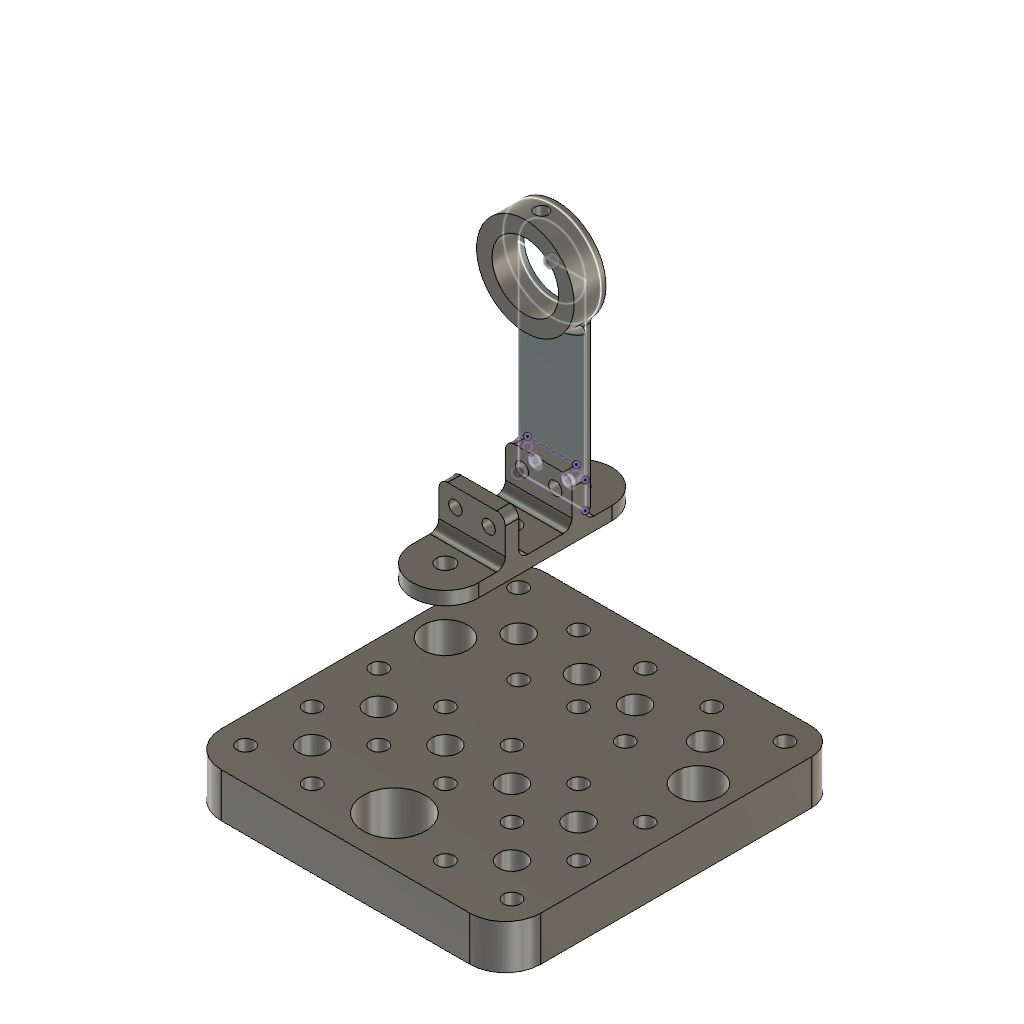
kobra2-neo-pen-holder (Autodesk Fusion 360 design; units mm, degrees)
Autodesk Fusion 360 part; units mm, degrees
note: some values were not read from the file. Chosen so that the rebuilt part matches the saved one: that a step has no effect; which face or edge a step refers to. Set by a fixed rule: which sketch regions a step uses.
sketch "Plate_Base_Profile" plane through (0, 0, 0) normal (0, 0, 1) x (1, 0, 0)
  line L0 (0, 0) -> (30, 0) construction
  circle A0 centre (30, 0) radius 1.9
  line L1 (0, 150) -> (0, -150) construction
  line L2 (0, 0) -> (0, -18) construction
  line L3 (0, -18) -> (12, -18) construction
  circle A1 centre (12, -18) radius 1.9
  line L4 (0, 0) -> (28.5, 0) construction
  line L5 (28.5, 0) -> (28.5, -18) construction
  circle A2 centre (28.5, -18) radius 5
  line L6 (0, 0) -> (0, -58) construction
  circle A3 centre (0, -58) radius 7
  circle A4 centre (0, -58) radius 11 construction
  circle A5 centre (30, 0) radius 6
  line L7 (30, 0) -> (30, 6) construction
  line L8 (30, 0) -> (36, 0) construction
  line L9 (30, 6) -> (0, 6)
  line L10 (0, -69) -> (28, -69)
  line L11 (36, 0) -> (36, -61)
  circle A6 centre (0, -58) radius 7
  line L12 (-30, 0) -> (-30, 6) construction
  circle A7 centre (-12, -18) radius 1.9
  circle A8 centre (-30, 0) radius 6
  line L13 (-30, 6) -> (0, 6)
  line L14 (0, 0) -> (-30, 0) construction
  circle A9 centre (0, -58) radius 11 construction
  line L15 (0, -69) -> (-28, -69)
  circle A10 centre (-30, 0) radius 1.9
  line L16 (0, 0) -> (-28.5, 0) construction
  line L17 (-28.5, 0) -> (-28.5, -18) construction
  circle A11 centre (-28.5, -18) radius 5
  line L18 (0, 0) -> (0, -18) construction
  line L19 (-36, 0) -> (-36, -61)
  line L20 (0, 0) -> (0, -58) construction
  line L21 (0, -18) -> (-12, -18) construction
  line L22 (-30, 0) -> (-36, 0) construction
  arc A12 (-36, -61) -> (-28, -69) centre (-28, -61) ccw
  arc A13 (28, -69) -> (36, -61) centre (28, -61) ccw
  dimension "d1" = 30
  dimension "d2" = 3.8
  dimension "d3" = 300
  dimension "d4" = 18
  dimension "d5" = 12
  dimension "d6" = 3.8
  dimension "d7" = 28.5
  dimension "d8" = 18
  dimension "d9" = 10
  dimension "d10" = 58
  dimension "d11" = 14
  dimension "d12" = 22
  dimension "d13" = 12
  dimension "d14" = 8
  constraint coincident L0.start L2.start
  constraint horizontal L0
  constraint coincident L0.end A0.centre
  constraint vertical L1
  constraint perpendicular L0 L2
  constraint perpendicular L2 L3
  constraint coincident L3.end A1.centre
  constraint perpendicular L1 L4
  constraint perpendicular L0 L5
  constraint coincident L5.end A2.centre
  constraint perpendicular L4 L6
  constraint coincident L6.end A3.centre
  constraint concentric A3 A4
  constraint concentric A0 A5
  constraint coincident A5 L7.end
  constraint perpendicular L0 L7
  constraint coincident A5 L8.end
  constraint perpendicular L7 L8
  constraint coincident L1 L9.end
  constraint tangent A5 L9
  constraint coincident A4 L10.start
  constraint coincident L1 L10.start
  constraint tangent A4 L10
  constraint perpendicular L1 L10
  constraint tangent A5 L11
  constraint symmetric L0.start L1 L2.start
  constraint symmetric L0.end L1 L12.start
  constraint symmetric A0 L1 A10
  constraint symmetric L1 L2.end L3.start
  constraint symmetric L1 L3.end A7.centre
  constraint symmetric L1 A1 A7
  constraint symmetric L1 L4.end L16.end
  constraint symmetric L1 L5.end L17.end
  constraint symmetric L1 A2 A11
  constraint symmetric L1 L6.end A3.centre
  constraint symmetric L1 A3 A6
  constraint symmetric L1 A4 A9
  constraint symmetric L1 A5 A8
  constraint symmetric L1 L7.end L12.end
  constraint symmetric L1 L8.end L19.start
  constraint symmetric L1 L9.end L13.end
  constraint symmetric L1 L10.start L15.start
  constraint tangent L19 A12
  constraint tangent L15 A12
  constraint tangent L10 A13
  constraint tangent L11 A13
  constraint equal A12 A13
  constraint tangent A4 L15
  constraint tangent A8 L19
  constraint midpoint L0.start L1
  measures "d1" distance of L0.start L0.end
  measures "d2" diameter of A0
  measures "d3" distance of L1.start L1.end
  measures "d4" distance of L0.start L2.end
  measures "d5" distance of L2.end L3.end
  measures "d6" diameter of A1
  measures "d7" distance of L0.start L4.end
  measures "d8" distance of L4.end L5.end
  measures "d9" diameter of A2
  measures "d10" distance of L0.start L6.end
  measures "d11" diameter of A3
  measures "d12" diameter of A4
  measures "d13" diameter of A5
  measures "d14" radius of A12
extrude "Plate_Base" add sketch "Plate_Base_Profile" along normal blind 10 makes body 1
sketch "Grid_Hole_Seed" plane through (0, 0, 10) normal (0, 0, 1) x (-1, 0, 0)
  circle A0 centre (28.5, 18) radius 5
  circle A1 centre (-30, 0) radius 1.9
  circle A2 centre (30, 0) radius 1.9
  circle A3 centre (12, 18) radius 1.9
  circle A4 centre (0, 58) radius 7
  circle A5 centre (-28.5, 18) radius 5
  circle A6 centre (-12, 18) radius 1.9
  line L0 (28, 69) -> (-28, 69)
  arc A7 (-28, 69) -> (-36, 61) centre (-28, 61) ccw
  line L1 (-36, 61) -> (-36, 0)
  arc A8 (-36, 0) -> (-30, -6) centre (-30, 0) ccw
  line L2 (-30, -6) -> (30, -6)
  arc A9 (30, -6) -> (36, 0) centre (30, 0) ccw
  line L3 (36, 0) -> (36, 61)
  arc A10 (36, 61) -> (28, 69) centre (28, 61) ccw
  line L4 (0, -6) -> (0, 69) construction
  circle A11 centre (0, 31.5) radius 1.9
  dimension "d19" = 3.8
  constraint midpoint L2 L4.start
  constraint coincident L0 L4.end
  constraint perpendicular L0 L4
  constraint midpoint L4 A11.centre
  measures "d19" diameter of A11
extrude "Grid_Hole_Cut" cut sketch "Grid_Hole_Seed" against normal through all contours A11 bodies 1
pattern_linear "Grid_Hole_Pattern" [no effect]
sketch "Mounting_Holes" plane through (0, 0, 10) normal (0, 0, 1) x (-1, 0, 0)
  circle A0 centre (0, 31.5) radius 1.9
  circle A1 centre (28.5, 18) radius 5
  circle A2 centre (-30, 0) radius 1.9
  circle A3 centre (30, 0) radius 1.9
  circle A4 centre (12, 18) radius 1.9
  circle A5 centre (0, 58) radius 7
  circle A6 centre (-28.5, 18) radius 5
  circle A7 centre (-12, 18) radius 1.9
  line L0 (28, 69) -> (-28, 69)
  arc A8 (-28, 69) -> (-36, 61) centre (-28, 61) ccw
  line L1 (-36, 61) -> (-36, 0)
  arc A9 (-36, 0) -> (-30, -6) centre (-30, 0) ccw
  line L2 (-30, -6) -> (30, -6)
  arc A10 (30, -6) -> (36, 0) centre (30, 0) ccw
  line L3 (36, 0) -> (36, 61)
  arc A11 (36, 61) -> (28, 69) centre (28, 61) ccw
  circle A12 centre (-30, 61.5) radius 1.9
  circle A13 centre (-30, 46.5) radius 1.9
  circle A14 centre (-30, 31.5) radius 1.9
  circle A15 centre (-15, 61.5) radius 1.9
  circle A16 centre (-15, 46.5) radius 1.9
  circle A17 centre (-15, 31.5) radius 1.9
  circle A18 centre (-15, 1.5) radius 1.9
  circle A19 centre (0, 46.5) radius 1.9
  circle A20 centre (0, 16.5) radius 1.9
  circle A21 centre (0, 1.5) radius 1.9
  circle A22 centre (15, 61.5) radius 1.9
  circle A23 centre (15, 46.5) radius 1.9
  circle A24 centre (15, 31.5) radius 1.9
  circle A25 centre (15, 1.5) radius 1.9
  circle A26 centre (30, 61.5) radius 1.9
  circle A27 centre (30, 46.5) radius 1.9
  circle A28 centre (30, 31.5) radius 1.9
  line L4 (15, 31.5) -> (30, 46.5) construction
  line L5 (30, 46.5) -> (30, 31.5) construction
  line L6 (30, 31.5) -> (15, 46.5) construction
  line L7 (15, 46.5) -> (0, 31.5) construction
  line L8 (0, 31.5) -> (-15, 46.5) construction
  line L9 (-15, 46.5) -> (-29.5655, 31.9345) construction
  line L10 (-29.5655, 31.9345) -> (-30, 46.5) construction
  line L11 (-30, 46.5) -> (-15, 31.5) construction
  line L12 (-15, 31.5) -> (0, 46.5) construction
  line L13 (0, 46.5) -> (15, 31.5) construction
  line L14 (0, 1.5) -> (12, 18) construction
  line L15 (0, 1.5) -> (-12, 18) construction
  line L16 (-12, 18) -> (-30, 0) construction
  line L17 (12, 18) -> (30, 0) construction
  line L18 (30, 46.5) -> (30, 61.5) construction
  line L19 (30, 61.5) -> (15, 46.5) construction
  line L20 (30, 46.5) -> (15, 61.5) construction
  line L21 (-15, 61.5) -> (-30, 46.5) construction
  line L22 (-30, 61.5) -> (-15, 46.5) construction
  circle A29 centre (22.5, 39) radius 3
  circle A30 centre (7.5, 39) radius 3
  circle A31 centre (-7.5, 39) radius 3
  circle A32 centre (-22.5, 39) radius 3
  circle A33 centre (22.5, 54) radius 3
  circle A34 centre (-22.5, 54) radius 3
  circle A35 centre (21, 9) radius 3
  circle A36 centre (6, 9.75) radius 3
  circle A37 centre (-6, 9.75) radius 3
  circle A38 centre (-21, 9) radius 3
  dimension "d26" = 6
  dimension "d27" = 6
  dimension "d28" = 6
  dimension "d29" = 6
  dimension "d30" = 6
  dimension "d31" = 6
  dimension "d32" = 6
  dimension "d33" = 6
  dimension "d34" = 6
  dimension "d35" = 6
  constraint coincident A24.centre L4.start
  constraint coincident A27.centre L4.end
  constraint coincident A28.centre L5.end
  constraint coincident A23.centre L6.end
  constraint coincident A0.centre L7.end
  constraint coincident A16.centre L8.end
  constraint perpendicular L8 L9
  constraint coincident A13.centre L10.end
  constraint coincident A17.centre L11.end
  constraint coincident A19.centre L12.end
  constraint coincident A21.centre L14.start
  constraint coincident A4.centre L14.end
  constraint coincident A7.centre L15.end
  constraint coincident A2.centre A9.centre
  constraint coincident A3.centre A10.centre
  constraint coincident A26.centre L18.end
  constraint coincident A22.centre L20.end
  constraint coincident A15.centre L21.start
  constraint coincident A12.centre L22.start
  constraint midpoint L4 A29.centre
  constraint midpoint L13 A30.centre
  constraint midpoint L12 A31.centre
  constraint midpoint L11 A32.centre
  constraint midpoint L19 A33.centre
  constraint midpoint L21 A34.centre
  constraint midpoint L17 A35.centre
  constraint midpoint L14 A36.centre
  constraint midpoint L15 A37.centre
  constraint midpoint L16 A38.centre
  measures "d26" diameter of A29
  measures "d27" diameter of A30
  measures "d28" diameter of A31
  measures "d30" diameter of A33
  measures "d32" diameter of A35
  measures "d33" diameter of A36
  measures "d34" diameter of A37
  measures "d35" diameter of A38
extrude "Mounting_Holes_Cut" cut sketch "Mounting_Holes" against normal through all contours A12 | A13 | A14 | A15 | A16 | A17 | A18 | A19 | A20 | A21 | A22 | A23 | A24 | A25 | A26 | A27 | A28 | A29 | A30 | A31 | A32 | A33 | A34 | A35 | A36 | A37 | A38 bodies 1
ref_plane "WorkPlane1" through (0, -31.5, 50) normal (0, 0, 1) x (1, 0, 0)
sketch "Pen_Base_Profile" plane through (0, 0, 50) normal (0, 0, 1) x (1, 0, 0)
  circle A0 centre (-30, -31.5) radius 1.9
  circle A1 centre (-30, -46.5) radius 1.9
  circle A2 centre (-30, -61.5) radius 1.9
  circle A3 centre (-15, -1.5) radius 1.9
  circle A4 centre (-15, -31.5) radius 1.9
  circle A5 centre (-15, -46.5) radius 1.9
  circle A6 centre (-15, -61.5) radius 1.9
  circle A7 centre (0, -1.5) radius 1.9
  circle A8 centre (0, -16.5) radius 1.9
  circle A9 centre (0, -46.5) radius 1.9
  circle A10 centre (15, -1.5) radius 1.9
  circle A11 centre (15, -31.5) radius 1.9
  circle A12 centre (15, -46.5) radius 1.9
  circle A13 centre (15, -61.5) radius 1.9
  circle A14 centre (30, -31.5) radius 1.9
  circle A15 centre (30, -46.5) radius 1.9
  circle A16 centre (30, -61.5) radius 1.9
  arc A17 (36, 0) -> (30, 6) centre (30, 0) ccw
  line L0 (30, 6) -> (-30, 6)
  arc A18 (-30, 6) -> (-36, 0) centre (-30, 0) ccw
  line L1 (-36, 0) -> (-36, -61)
  arc A19 (-36, -61) -> (-28, -69) centre (-28, -61) ccw
  line L2 (-28, -69) -> (28, -69)
  arc A20 (28, -69) -> (36, -61) centre (28, -61) ccw
  line L3 (36, -61) -> (36, 0)
  circle A21 centre (30, 0) radius 1.9
  circle A22 centre (-12, -18) radius 1.9
  circle A23 centre (-28.5, -18) radius 5
  circle A24 centre (28.5, -18) radius 5
  circle A25 centre (0, -58) radius 7
  circle A26 centre (12, -18) radius 1.9
  circle A27 centre (-30, 0) radius 1.9
  circle A28 centre (0, -31.5) radius 1.9
  circle A29 centre (-22.5, -54) radius 3
  circle A30 centre (22.5, -54) radius 3
  circle A31 centre (-6, -9.75) radius 3
  circle A32 centre (6, -9.75) radius 3
  circle A33 centre (7.5, -39) radius 3
  circle A34 centre (-22.5, -39) radius 3
  circle A35 centre (22.5, -39) radius 3
  circle A36 centre (-21, -9) radius 3
  circle A37 centre (21, -9) radius 3
  circle A38 centre (-7.5, -39) radius 3
  circle A39 centre (0, -16.5) radius 7.5
  circle A40 centre (0, -46.5) radius 7.5
  line L4 (0, -46.5) -> (-7.5, -46.5) construction
  line L5 (-7.5, -16.5) -> (0, -16.5) construction
  line L6 (-7.5, -16.5) -> (-7.5, -46.5)
  line L7 (0, -16.5) -> (7.5, -16.5) construction
  line L8 (0, -46.5) -> (7.5, -46.5) construction
  line L9 (7.5, -16.5) -> (7.5, -46.5)
  circle A41 centre (0, -16.5) radius 2
  circle A42 centre (0, -46.5) radius 2
  dimension "d62" = 15
  dimension "d63" = 15
  dimension "d64" = 4
  dimension "d65" = 4
  constraint concentric A8 A39
  constraint concentric A9 A40
  constraint coincident A9.centre A40.centre
  constraint coincident A40 L4.end
  constraint horizontal L4
  constraint coincident A39 L5.start
  constraint coincident A8.centre A39.centre
  constraint tangent A40 L6
  constraint coincident A39 L7.end
  constraint parallel L5 L7
  constraint coincident A40 L8.end
  constraint parallel L4 L8
  constraint concentric A8 A41
  constraint concentric A40 A42
  measures "d62" diameter of A39
  measures "d63" diameter of A40
  measures "d64" diameter of A41
  measures "d65" diameter of A42
extrude "Pen_Base_Plate" add sketch "Pen_Base_Profile" along normal blind 3 separate body contours A25 A40 | A25 A40 | A33 A38 A39 A40 L6 L9 | A33 L9 | A38 L6 | A31 A32 A39 | A32 A39 | A31 A39 picked at (0, -52.9878) picked at (-3.6256, -49.8497) picked at (6.2303, -39.7331) picked at (-5.9134, -39.6549) picked at (4.6509, -11.2678) picked at (-4.6663, -11.2812) makes body 2
sketch "Pen_Base_Reinforcements" plane through (0, 0, 53) normal (0, 0, 1) x (-1, 0, 0)
  circle A0 centre (0, 46.5) radius 2
  circle A1 centre (0, 16.5) radius 2
  circle A2 centre (0, 31.5) radius 1.9
  line L0 (7.5, 16.5) -> (7.5, 46.5)
  arc A3 (7.5, 46.5) -> (-7.5, 46.5) centre (0, 46.5) ccw
  line L1 (-7.5, 46.5) -> (-7.5, 16.5)
  arc A4 (-7.5, 16.5) -> (7.5, 16.5) centre (0, 16.5) ccw
  line L2 (0, 16.5) -> (0, 31.5) construction
  line L3 (0, 31.5) -> (0, 46.5) construction
  line L4 (0, 39) -> (7.5, 39) construction
  line L5 (0, 24) -> (7.5, 24) construction
  line L6 (0, 24) -> (-7.5, 24) construction
  line L7 (0, 39) -> (-7.5, 39) construction
  line L8 (-7.5, 40.5) -> (7.5, 40.5)
  line L9 (7.5, 40.5) -> (7.5, 37.5)
  line L10 (7.5, 37.5) -> (-7.5, 37.5)
  line L11 (-7.5, 37.5) -> (-7.5, 40.5)
  line L12 (-7.5, 40.5) -> (7.5, 37.5) construction
  line L13 (7.5, 40.5) -> (-7.5, 37.5) construction
  line L14 (-7.5, 25.5) -> (7.5, 25.5)
  line L15 (7.5, 25.5) -> (7.5, 22.5)
  line L16 (7.5, 22.5) -> (-7.5, 22.5)
  line L17 (-7.5, 22.5) -> (-7.5, 25.5)
  line L18 (-7.5, 25.5) -> (7.5, 22.5) construction
  line L19 (7.5, 25.5) -> (-7.5, 22.5) construction
  point P0 (0, 39)
  point P1 (0, 24)
  dimension "d68" = 3
  dimension "d69" = 3
  dimension "d119" = 15
  constraint coincident A1.centre A4.centre
  constraint coincident A2.centre L2.end
  constraint coincident A0.centre A3.centre
  constraint midpoint L3 P0
  constraint coincident L0 L4.end
  constraint perpendicular L0 L4
  constraint midpoint L2 P1
  constraint coincident L0 L5.end
  constraint perpendicular L0 L5
  constraint coincident L1 L6.end
  constraint perpendicular L1 L6
  constraint coincident L1 L7.end
  constraint perpendicular L1 L7
  constraint horizontal L8
  constraint perpendicular L8 L9
  constraint parallel L8 L10
  constraint parallel L9 L11
  constraint coincident L12 P0
  constraint coincident L13 P0
  constraint coincident P0 L4.start
  constraint horizontal L14
  constraint perpendicular L14 L15
  constraint parallel L14 L16
  constraint parallel L15 L17
  constraint coincident L18 P1
  constraint coincident L19 P1
  constraint coincident P1 L5.start
  constraint equal L8 L14
  measures "d68" distance of L8.end L9.end
  measures "d69" distance of L14.end L15.end
  measures "d119" horizontal distance of L8.start L8.end
extrude "Pen_Base_Reinforcement" add sketch "Pen_Base_Reinforcements" along normal blind 10 contours L0 L1 L14 L15 L16 L17 | L0 L1 L8 L9 L10 L11 bodies 2
fillet "Pen_Base_Fillet_A" radius 2 4 edges at (0, -22.5, 53) (0, -37.5, 53) (0, -25.5, 53) (0, -40.5, 53) on bodies 2
fillet "Pen_Base_Fillet_B" radius 2 4 edges at (-7.5, -24, 63) (7.5, -24, 63) (-7.5, -39, 63) (7.5, -39, 63) on bodies 2
sketch "Insert_Pilot_Holes" plane through (0, -22.5, 0) normal (0, 1, 0) x (-1, 0, 0)
  arc A0 (-5.5, 63) -> (-7.5, 61) centre (-5.5, 61) ccw
  line L0 (-7.5, 61) -> (-7.5, 55)
  line L1 (-7.5, 55) -> (7.5, 55)
  line L2 (7.5, 55) -> (7.5, 61)
  arc A1 (7.5, 61) -> (5.5, 63) centre (5.5, 61) ccw
  line L3 (5.5, 63) -> (-5.5, 63)
  line L4 (7.5, 53) -> (7.5, 55)
  line L5 (7.5, 55) -> (-7.5, 55)
  line L6 (-7.5, 55) -> (-7.5, 53)
  line L7 (-7.5, 53) -> (7.5, 53)
  line L8 (0, 53) -> (0, 63) construction
  line L9 (0, 55) -> (0, 59) construction
  line L10 (0, 59) -> (3.75, 59) construction
  line L11 (0, 59) -> (-3.75, 59) construction
  circle A2 centre (3.75, 59) radius 1.5
  circle A3 centre (-3.75, 59) radius 1.5
  dimension "d76" = 4
  dimension "d77" = 3.75
  dimension "d78" = 3.75
  dimension "d79" = 3
  dimension "d80" = 3
  constraint midpoint L7 L8.start
  constraint midpoint L3 L8.end
  constraint midpoint L5 L9.start
  constraint perpendicular L3 L9
  constraint perpendicular L2 L10
  constraint perpendicular L8 L11
  constraint coincident L10.end A2.centre
  constraint coincident L11.end A3.centre
  measures "d76" distance of L9.start L9.end
  measures "d77" distance of L9.end L10.end
  measures "d78" distance of L9.end L11.end
  measures "d79" diameter of A2
  measures "d80" diameter of A3
extrude "Insert_Pilot_Holes_Cut" cut sketch "Insert_Pilot_Holes" against normal up to surface (18 mm away) contours A2 | A3 bodies 2
sketch "Flex_Link_And_Pen_Clamp_Profile" plane through (0, -22.5, 0) normal (0, 1, 0) x (-1, 0, 0)
  arc A0 (-5.5, 63) -> (-7.5, 61) centre (-5.5, 61) ccw
  line L0 (-7.5, 61) -> (-7.5, 55)
  line L1 (-7.5, 55) -> (7.5, 55)
  line L2 (7.5, 55) -> (7.5, 61)
  arc A1 (7.5, 61) -> (5.5, 63) centre (5.5, 61) ccw
  line L3 (5.5, 63) -> (-5.5, 63)
  line L4 (7.5, 55) -> (-7.5, 55)
  line L5 (-7.5, 55) -> (-7.5, 100)
  line L6 (-7.5, 100) -> (7.5, 100)
  line L7 (7.5, 100) -> (7.5, 55)
  circle A2 centre (-3.75, 59) radius 1.3
  circle A3 centre (3.75, 59) radius 1.3
  circle A4 centre (0, 100) radius 11
  circle A5 centre (0, 100) radius 7.5
  circle A6 centre (3.75, 59) radius 1.5
  circle A7 centre (-3.75, 59) radius 1.5
  dimension "d83" = 15
  dimension "d84" = 45
  dimension "d85" = 2.6
  dimension "d86" = 2.6
  dimension "d87" = 22
  dimension "d121" = 15
  constraint horizontal L4
  constraint vertical L5
  constraint horizontal L6
  constraint vertical L7
  constraint coincident L1.end L2.start
  constraint midpoint L6 A4.centre
  constraint concentric A4 A5
  constraint concentric A2 A7
  constraint concentric A3 A6
  measures "d83" distance of L1.end L0.end
  measures "d84" distance of L1.end L6.end
  measures "d85" diameter of A2
  measures "d86" diameter of A3
  measures "d87" diameter of A4
  measures "d121" diameter of A5
extrude "Flex_Link_Base" add sketch "Flex_Link_And_Pen_Clamp_Profile" along normal blind 1.2 separate body contours A0 L0 L1 L2 A1 L3 L4 L5 L7 | A0 A1 L3 L5 L7 A4 | L5 L7 A4 A5 | L5 L7 A4 A5 | A6 | A7 makes body 3
extrude "Pen_Clamp_Reinforcement" add sketch "Flex_Link_And_Pen_Clamp_Profile" against normal blind 6 contours L5 L7 A4 A5 | L5 L7 A4 A5 bodies 3
fillet "Pen_Clamp_Fillet" radius 2 3 edges at (-7.5, -21.9, 91.9533) (0, -22.5, 89) (7.5, -21.9, 91.9533) on bodies 3
ref_plane "WorkPlane2" through (0, 0, 120) normal (0, 0, 1) x (1, 0, 0)
sketch "Clamp_Screw_Insert_Hole" plane through (0, 0, 120) normal (0, 0, 1) x (1, 0, 0)
  line L0 (8.0385, -24.5) -> (8.0385, -21.3)
  line L1 (11, -21.3) -> (-11, -21.3)
  line L2 (-8.0385, -21.3) -> (-8.0385, -24.5)
  line L3 (8.0385, -24.5) -> (-8.0385, -24.5)
  line L4 (-11, -28.5) -> (11, -28.5)
  line L5 (-11, -28.5) -> (11, -21.3) construction
  line L6 (11, -28.5) -> (-11, -21.3) construction
  circle A0 centre (0, -24.9) radius 1.5
  dimension "d96" = 3
  constraint coincident L4.start L5.start
  constraint coincident L1.start L5.end
  constraint coincident L4.end L6.start
  constraint coincident L1.end L6.end
  constraint midpoint L6 A0.centre
  measures "d96" diameter of A0
extrude "Clamp_Screw_Insert_Hole_Cut" cut sketch "Clamp_Screw_Insert_Hole" along normal up to surface contours L3 A0 | L3 A0 end surface at (-7.4907, -21.7, 99.6262) on bodies 3 bodies 3
equation "d1 = outerSmallHoleX"
equation "d2 = gridHoleDiameter"
equation "d3 = symmetryAxisLength"
equation "d4 = featureRowY"
equation "d5 = innerSmallHoleX"
equation "d6 = gridHoleDiameter"
equation "d7 = largeSideHoleX"
equation "d8 = featureRowY"
equation "d9 = largeSideHoleDiameter"
equation "d10 = centerLargeHoleY"
equation "d11 = centerLargeHoleDiameter"
equation "d12 = centerLargeHoleDiameter + 2 * centerLargeHoleEdgeClearance"
equation "d13 = 2 * topCornerRadius"
equation "d14 = bottomCornerRadius"
equation "d17 = plateThickness"
equation "d19 = gridHoleDiameter"
equation "d22 = gridCountY"
equation "d23 = gridCountX"
equation "d24 = gridPatternExtentY"
equation "d25 = gridPatternExtentX"
equation "d26 = mountHoleDiameter"
equation "d27 = mountHoleDiameter"
equation "d28 = mountHoleDiameter"
equation "d29 = mountHoleDiameter"
equation "d30 = mountHoleDiameter"
equation "d31 = mountHoleDiameter"
equation "d32 = mountHoleDiameter"
equation "d33 = mountHoleDiameter"
equation "d34 = mountHoleDiameter"
equation "d35 = mountHoleDiameter"
equation "plateThickness = 10 mm" comment "Main printed plate thickness"
equation "gridHoleDiameter = 3.8 mm" comment "Diameter of the patterned grid hole seed"
equation "gridCountX = 5" comment "Number of grid instances across X"
equation "gridCountY = 5" comment "Number of grid instances across Y"
equation "gridPatternExtentX = 30 mm" comment "Total symmetric X extent of the grid pattern (not pitch)"
equation "gridPatternExtentY = 30 mm" comment "Total symmetric Y extent of the grid pattern (not pitch)"
equation "mountHoleDiameter = 6 mm" comment "Common diameter for the ten mounting holes"
equation "symmetryAxisLength = 300 mm" comment "Construction axis length used by symmetry constraints in Plate_Base_Profile"
equation "outerSmallHoleX = 30 mm" comment "X offset of the outer Ã3.8 hole / upper corner center"
equation "featureRowY = 18 mm" comment "Y offset of the secondary feature row"
equation "innerSmallHoleX = 12 mm" comment "X offset of the inner Ã3.8 hole on the secondary row"
equation "largeSideHoleX = 28.5 mm" comment "X offset of the Ã10 side hole"
equation "largeSideHoleDiameter = 10 mm" comment "Diameter of the side large hole"
equation "centerLargeHoleY = 58 mm" comment "Y offset of the lower/central large hole"
equation "centerLargeHoleDiameter = 14 mm" comment "Diameter of the lower/central large hole"
equation "centerLargeHoleEdgeClearance = 4 mm" comment "Minimum material from the Ã14 hole to the tangent bottom edge"
equation "topCornerRadius = 6 mm" comment "Radius of the upper outer corners"
equation "bottomCornerRadius = 8 mm" comment "Radius of the lower outer corners"
equation "plateWidth = 2 * ( outerSmallHoleX + topCornerRadius )" comment "Derived overall plate width"
equation "plateHeight = topCornerRadius + centerLargeHoleY + centerLargeHoleDiameter / 2 + centerLargeHoleEdgeClearance" comment "Derived overall plate height"
equation "gridPitchX = gridPatternExtentX / ( gridCountX - 1 )" comment "Derived center-to-center pitch across X"
equation "gridPitchY = gridPatternExtentY / ( gridCountY - 1 )" comment "Derived center-to-center pitch across Y"
equation "d60 = penMountPlaneOffset"
equation "d62 = penBaseBossDiameter"
equation "d63 = penBaseBossDiameter"
equation "d64 = penBaseMountHoleDiameter"
equation "d65 = penBaseMountHoleDiameter"
equation "d66 = penBaseThickness"
equation "d68 = penBaseTabHeight"
equation "d69 = penBaseTabHeight"
equation "d70 = penBaseReinforcementHeight"
equation "d73 = penBaseFilletRadius"
equation "d75 = penBaseFilletRadius"
equation "d76 = insertRowOffset"
equation "d77 = linkFastenerSpacing / 2"
equation "d78 = linkFastenerSpacing / 2"
equation "d79 = insertPilotDiameter"
equation "d80 = insertPilotDiameter"
equation "d83 = flexLinkWidth"
equation "d84 = flexLinkLength"
equation "d85 = linkScrewClearanceDiameter"
equation "d86 = linkScrewClearanceDiameter"
equation "d87 = penClampOuterDiameter"
equation "d88 = flexLinkThickness"
equation "d90 = -penClampDepth"
equation "d93 = penClampFilletRadius"
equation "d94 = clampScrewSketchPlaneOffset"
equation "d96 = insertPilotDiameter"
equation "penMountPlaneOffset = 40 mm" comment "Offset from mounting plate reference face to pen-base sketch plane."
equation "penBaseBossDiameter = 15 mm" comment "Outer diameter of the two pen-mount base bosses."
equation "penBaseMountHoleDiameter = 4 mm" comment "Mounting-hole diameter in the pen-mount base."
equation "penBaseThickness = 3 mm" comment "Base plate thickness of the pen-mount adapter."
equation "penBaseTabHeight = 3 mm" comment "Height of each reinforcing tab in the pen-mount base sketch."
equation "penBaseReinforcementHeight = 10 mm" comment "Extrusion height of the pen-mount base reinforcement."
equation "penBaseFilletRadius = 2 mm" comment "Fillet radius used on the pen-mount base."
equation "insertPilotDiameter = 3 mm" comment "Pilot bore for the 3.4 mm press/heat-set insert."
equation "insertNominalOD = 3.4 mm" comment "Reference outside diameter of the physical insert; not a cut diameter."
equation "insertRowOffset = 4 mm" comment "Vertical offset locating the insert row in the base."
equation "linkFastenerSpacing = 7.5 mm" comment "Center-to-center spacing of the pair of link fasteners."
equation "flexLinkWidth = 15 mm" comment "Width of the flexible PLA link."
equation "flexLinkLength = 45 mm" comment "Functional length of the flexible PLA link."
equation "linkScrewClearanceDiameter = 2.6 mm" comment "Clearance hole for the approximately 2.44 mm link screw."
equation "penClampOuterDiameter = 22 mm" comment "Outer diameter of the pen clamp ring."
equation "flexLinkThickness = 1.2 mm" comment "Printed thickness of the flexible PLA link."
equation "penClampDepth = 6 mm" comment "Additional rigid clamp depth beyond the flexible-link thickness."
equation "penClampFilletRadius = 2 mm" comment "Fillet radius on the pen clamp transition."
equation "clampScrewSketchPlaneOffset = 120 mm" comment "Reference-plane offset used for the pen clamp insert/screw pilot."
equation "penBaseWidth = 15 mm" comment "Overall width of the pen-mount base and reinforcement tabs."
equation "d119 = penBaseWidth"
equation "penClampBoreDiameter = 15 mm" comment "Nominal diameter of the pen bore; independent of flexible-link width."
equation "d121 = penClampBoreDiameter"
named bodies: "Mounting_Plate", "Pen_Mount_Base", "Flex_Link_Pen_Holder"
